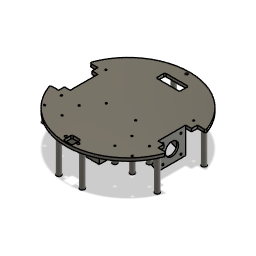
podvozek9_line_follow v3 (Autodesk Fusion 360 design; units mm, degrees)
Autodesk Fusion 360 part; units mm, degrees
sketch "zakladna" plane through (0, 0, 0) normal (0, 1, 0) x (1, 0, 0)
  line L0 (-40.0372, -23.4927) -> (-85, -23.4927)
  line L1 (39.9628, -23.4927) -> (85, -23.4927)
  line L2 (-85, 23.5073) -> (-40.0372, 23.5073)
  line L3 (85, 23.5073) -> (39.9628, 23.5073)
  line L4 (1.75, 0) -> (22.5, 0)
  line L5 (-96.7123, 33.4364) -> (-85, 33.4364)
  line L6 (-85, 33.4364) -> (-85, 23.5073)
  line L7 (-96.7154, -33.4277) -> (-85, -33.4277)
  line L8 (-85, -33.4277) -> (-85, -23.4927)
  line L9 (96.7154, -33.4277) -> (85, -33.4277)
  line L10 (85, -33.4277) -> (85, -23.4927)
  line L11 (96.7123, 33.4364) -> (85, 33.4364)
  line L12 (85, 33.4364) -> (85, 23.5073)
  arc A0 (-98.5934, -36.1156) -> (98.5934, -36.1156) centre (0, 0) ccw
  arc A1 (-96.7154, -33.4277) -> (-98.5934, -36.1156) centre (-96.7154, -35.4277) ccw
  arc A2 (-98.5902, 36.1245) -> (-96.7123, 33.4364) centre (-96.7123, 35.4364) ccw
  arc A3 (96.7123, 33.4364) -> (98.5902, 36.1245) centre (96.7123, 35.4364) ccw
  arc A4 (98.5934, -36.1156) -> (96.7154, -33.4277) centre (96.7154, -35.4277) ccw
  line L13 (0, -1.75) -> (0, -22.5)
  line L14 (39.9628, -23.4927) -> (34.9628, -23.4927)
  line L15 (34.9628, -23.4927) -> (34.9628, 23.5073)
  line L16 (34.9628, 23.5073) -> (39.9628, 23.5073)
  line L17 (-40.0372, -23.4927) -> (-35.0372, -23.4927)
  line L18 (-35.0372, -23.4927) -> (-35.0372, 23.5073)
  line L19 (-35.0372, 23.5073) -> (-40.0372, 23.5073)
  line L20 (0, -20) -> (0, -2.5)
  line L21 (2.5, 0) -> (20, 0)
  line L22 (0, 105) -> (0, -105) construction
  line L23 (-105, 0) -> (104.2756, 0.0073) construction
  line L24 (-40, -12.9977) -> (44.2998, -12.9948) construction
  circle A5 centre (-25, -11.9963) radius 1.4
  circle A6 centre (-75, 37.0037) radius 1.4
  circle A7 centre (25, -11.9963) radius 1.4
  circle A8 centre (75, 37.0037) radius 1.4
  line L25 (-20, 83.0037) -> (20, 83.0037)
  line L26 (20, 83.0037) -> (20, 68.0037)
  line L27 (20, 68.0037) -> (-20, 68.0037)
  line L28 (-20, 68.0037) -> (-20, 83.0037)
  circle A9 centre (-10.5, -95.4967) radius 2.1
  circle A10 centre (10.5, -95.4967) radius 2.1
  line L29 (-5.5, -87.9967) -> (5.5, -87.9967)
  line L30 (7.5, -89.9967) -> (7.5, -100.9967)
  line L31 (5.5, -102.9967) -> (-5.5, -102.9967)
  line L32 (-7.5, -100.9967) -> (-7.5, -89.9967)
  line L33 (-10.5, -95.4967) -> (10.5, -95.4967) construction
  arc A11 (-5.5, -87.9967) -> (-7.5, -89.9967) centre (-5.5, -89.9967) ccw
  arc A12 (7.5, -89.9967) -> (5.5, -87.9967) centre (5.5, -89.9967) ccw
  arc A13 (5.5, -102.9967) -> (7.5, -100.9967) centre (5.5, -100.9967) ccw
  arc A14 (-7.5, -100.9967) -> (-5.5, -102.9967) centre (-5.5, -100.9967) ccw
  arc A15 (98.5902, 36.1245) -> (15, 103.923) centre (0, 0) ccw
  arc A16 (-15, 103.923) -> (-98.5902, 36.1245) centre (0, 0) ccw
  line L34 (75, -38.4927) -> (45, -38.4927) construction
  line L35 (45, -38.4927) -> (45, -67.4927) construction
  line L36 (45, -67.4927) -> (75, -67.4927) construction
  line L37 (75, -67.4927) -> (75, -38.4927) construction
  circle A17 centre (45, -38.4927) radius 1.45
  circle A18 centre (75, -38.4927) radius 1.45
  circle A19 centre (45, -67.4927) radius 1.45
  circle A20 centre (75, -67.4927) radius 1.45
  circle A21 centre (-45, -38.4927) radius 1.45
  circle A22 centre (-75, -38.4927) radius 1.45
  circle A23 centre (-75, -67.4927) radius 1.45
  circle A24 centre (-45, -67.4927) radius 1.45
  line L38 (34.9628, -23.4927) -> (74.9628, -23.4927)
  line L39 (74.9628, -23.4927) -> (74.9628, 23.5073)
  line L40 (74.9628, 23.5073) -> (34.9628, 23.5073)
  line L41 (34.9628, 23.5073) -> (34.9628, -23.4927)
  line L42 (-35.0372, -23.4927) -> (-75.0372, -23.4927)
  line L43 (-75.0372, -23.4927) -> (-75.0372, 23.5073)
  line L44 (-75.0372, 23.5073) -> (-35.0372, 23.5073)
  line L45 (-35.0372, 23.5073) -> (-35.0372, -23.4927)
  arc A25 (15, 103.923) -> (-15, 103.923) centre (0, 0) ccw
  circle A26 centre (0, 100) radius 2.1
  point P0 (-82.0372, 22.8073)
  point P1 (-17.0372, -22.7927)
  point P2 (-0.0372, 0.0073)
  point P3 (81.9628, 22.8073)
  point P4 (-82.0372, -22.7927)
  point P5 (16.9628, 22.8073)
  point P6 (16.9628, 27.0073)
  point P7 (-17.0372, 27.0073)
  point P8 (81.9628, -22.7927)
  point P9 (16.9628, -22.7927)
  point P10 (16.9628, -26.9927)
  point P11 (-7.5, -87.9967)
  point P12 (7.5, -87.9967)
  point P13 (-7.5, -102.9967)
  dimension "d87" = 210
  dimension "d134" = 2
  dimension "d135" = 2
  dimension "d136" = 2
  dimension "d137" = 2
  dimension "d197" = 47
  dimension "d199" = 47
  dimension "d205" = 13
  dimension "d206" = 2.8
  dimension "d207" = 2.8
  dimension "d208" = 49
  dimension "d209" = 50
  dimension "d210" = 40
  dimension "d211" = 15
  dimension "d212" = 80
  dimension "d216" = 4.2
  dimension "d217" = 10.5
  dimension "d220" = 15
  dimension "d221" = 15
  dimension "d222" = 2
  dimension "d223" = 2
  dimension "d224" = 2
  dimension "d225" = 2
  dimension "d232" = 95.5
  dimension "d237" = 25
  dimension "d258" = 30
  dimension "d259" = 29
  dimension "d260" = 2.9
  dimension "d261" = 2.9
  dimension "d262" = 2.9
  dimension "d263" = 2.9
  dimension "d264" = 45
  dimension "d265" = 15
  dimension "d266" = 40
  dimension "d267" = 40
  dimension "d268" = 47
  dimension "d298" = 4.2
  dimension "d299" = 5
  constraint horizontal L2
  constraint horizontal L0
  constraint horizontal L3
  constraint horizontal L1
  constraint horizontal L5
  constraint vertical L6
  constraint horizontal L7
  constraint vertical L8
  constraint horizontal L9
  constraint vertical L10
  constraint horizontal L11
  constraint vertical L12
  constraint coincident A0.centre A15.centre
  constraint concentric A0 A15
  constraint tangent A0 A1
  constraint tangent L7 A1
  constraint tangent A2 A15
  constraint tangent L5 A2
  constraint tangent L11 A3
  constraint tangent A3 A15
  constraint tangent L9 A4
  constraint tangent A0 A4
  constraint horizontal L14
  constraint vertical L15
  constraint horizontal L16
  constraint horizontal L17
  constraint vertical L18
  constraint horizontal L19
  constraint midpoint A0 L22.end
  constraint parallel L20 L22
  constraint parallel L23 L24
  constraint symmetric L22 A5 A7
  constraint symmetric L22 A6 A8
  constraint horizontal L25
  constraint vertical L26
  constraint horizontal L27
  constraint vertical L28
  constraint symmetric L22 L26 L28
  constraint symmetric L22 A9 A10
  constraint horizontal L29
  constraint vertical L30
  constraint horizontal L31
  constraint vertical L32
  constraint symmetric L22 L30 L32
  constraint coincident A9.centre L33.start
  constraint coincident A10.centre L33.end
  constraint symmetric L29 L31 L33
  constraint coincident P11 L29
  constraint coincident P11 L32
  constraint tangent L29 A11
  constraint tangent L32 A11
  constraint coincident P12 L29
  constraint coincident P12 L30
  constraint tangent L29 A12
  constraint tangent L30 A12
  constraint tangent L30 A13
  constraint tangent L31 A13
  constraint coincident P13 L31
  constraint coincident P13 L32
  constraint tangent L31 A14
  constraint tangent L32 A14
  constraint concentric A15 A16
  constraint coincident L22.start A15
  constraint horizontal L34
  constraint vertical L35
  constraint horizontal L36
  constraint vertical L37
  constraint coincident L34.end L35.start
  constraint coincident L34.start L37.end
  constraint coincident L35.end L36.start
  constraint coincident L36.end L37.start
  constraint symmetric L22 A17 A21
  constraint symmetric L22 A18 A22
  constraint symmetric L22 A19 A24
  constraint symmetric L22 A20 A23
  constraint horizontal L38
  constraint vertical L39
  constraint horizontal L40
  constraint vertical L41
  constraint horizontal L42
  constraint vertical L43
  constraint horizontal L44
  constraint vertical L45
  constraint coincident L22.start A25
  constraint coincident L22 A26.centre
  measures "d87" diameter of A15
  measures "d134" radius of A1
  measures "d135" radius of A2
  measures "d136" radius of A3
  measures "d137" radius of A4
  measures "d197" distance of L1.start L3.end
  measures "d199" distance of L0.start L2.end
  measures "d205" distance of L23 L24
  measures "d206" diameter of A5
  measures "d207" diameter of A6
  measures "d208" vertical distance of A5.centre A6.centre
  measures "d209" horizontal distance of A5.centre A6.centre
  measures "d210" distance of L25.start L25.end
  measures "d211" distance of L25.start L27.end
  measures "d212" distance of A7.centre L27
  measures "d216" diameter of A9
  measures "d217" distance of L22 A9.centre
  measures "d220" distance of P11 P12
  measures "d221" distance of P11 P13
  measures "d222" radius of A11
  measures "d223" radius of A12
  measures "d224" radius of A13
  measures "d225" radius of A14
  measures "d232" distance of L23 A9.centre
  measures "d237" distance of L22 A5.centre
  measures "d258" distance of L34.start L34.end
  measures "d259" distance of L34.start L36.end
  measures "d260" diameter of A17
  measures "d261" diameter of A18
  measures "d262" diameter of A19
  measures "d263" diameter of A20
  measures "d264" distance of L22 L34.end
  measures "d265" distance of L1 L34.end
  measures "d266" distance of L14.end L38.end
  measures "d267" distance of L17.end L42.end
  measures "d268" distance of L17.end L18.end
  measures "d298" diameter of A26
  measures "d299" distance of L22.start A26.centre
extrude "Extrude23" add sketch "zakladna" along normal blind 5 contours L0 L1 L2 L3 L5 L6 L7 L8 L9 L10 L11 L12 A0 A1 A2 A3 A4 L14 L15 L16 L17 L18 L19 A15 A16 L38 L40 L41 L42 L44 L45 A25
sketch "beterka" plane through (0, 0, 0) normal (0, 1, 0) x (1, 0, 0)
  line L0 (-36, -25) -> (36, -25)
  line L1 (36, -25) -> (36, -85)
  line L2 (36, -85) -> (-36, -85)
  line L3 (-36, -85) -> (-36, -25)
  line L4 (0, 105) -> (0, -105)
  line L5 (2.5, 0) -> (20, 0)
  line L6 (37.5, -86.5) -> (-37.5, -86.5)
  line L7 (-37.5, -86.5) -> (-37.5, -23.5)
  line L8 (-37.5, -23.5) -> (37.5, -23.5)
  line L9 (37.5, -23.5) -> (37.5, -86.5)
  dimension "d228" = 72
  dimension "d229" = 60
  dimension "d230" = 25
  dimension "d231" = -1.5
  constraint horizontal L0
  constraint vertical L1
  constraint horizontal L2
  constraint vertical L3
  constraint symmetric L1 L3 L4
  measures "d228" distance of L0.start L0.end
  measures "d229" distance of L0.start L2.end
  measures "d230" distance of L0 L5
extrude "Extrude25" add sketch "beterka" against normal blind 17 contours L0 L2 L3 L4 L6 L7 L8 | L0 L1 L2 L4 L6 L8 L9
sketch "zvyseni" plane through (0, 0, 0) normal (0, 1, 0) x (1, 0, 0)
  circle A0 centre (25, -11.9963) radius 4
  circle A1 centre (25, -11.9963) radius 1.4
  circle A2 centre (-25, -11.9963) radius 1.4
  circle A3 centre (-25, -11.9963) radius 4
  circle A4 centre (75, 37.0037) radius 1.4
  circle A5 centre (75, 37.0037) radius 4
  circle A6 centre (-75, 37.0037) radius 1.4
  circle A7 centre (-75, 37.0037) radius 4
  line L0 (5, 90) -> (-5, 90)
  line L1 (-5, 90) -> (-5, 85)
  line L2 (-5, 85) -> (5, 85)
  line L3 (5, 85) -> (5, 90)
  point P0 (25, -11.9963)
  point P1 (-25, -11.9963)
  point P2 (75, 37.0037)
  point P3 (-75, 37.0037)
  dimension "d250" = 8
  dimension "d251" = 8
  dimension "d252" = 8
  dimension "d253" = 8
  constraint coincident P0 A0.centre
  constraint coincident P1 A2.centre
  constraint coincident P2 A4.centre
  constraint concentric A4 A5
  constraint coincident P3 A6.centre
  constraint concentric A6 A7
  constraint horizontal L0
  constraint vertical L1
  constraint horizontal L2
  constraint vertical L3
  measures "d250" diameter of A0
  measures "d251" diameter of A3
  measures "d252" diameter of A5
  measures "d253" diameter of A7
extrude "Extrude26" add sketch "zvyseni" against normal blind 1.6
sketch " motory_podklad" plane through (0, 5, 0) normal (0, 1, 0) x (-1, 0, 0)
  circle A0 centre (-45, 67.4927) radius 1.45
  circle A1 centre (-10.5, 95.4967) radius 2.1
  circle A2 centre (-75, 38.4927) radius 1.45
  arc A3 (5.5, 87.9967) -> (7.5, 89.9967) centre (5.5, 89.9967) ccw
  line L0 (5.5, 87.9967) -> (-5.5, 87.9967)
  arc A4 (-7.5, 89.9967) -> (-5.5, 87.9967) centre (-5.5, 89.9967) ccw
  line L1 (-7.5, 89.9967) -> (-7.5, 100.9967)
  arc A5 (-5.5, 102.9967) -> (-7.5, 100.9967) centre (-5.5, 100.9967) ccw
  line L2 (-5.5, 102.9967) -> (5.5, 102.9967)
  arc A6 (7.5, 100.9967) -> (5.5, 102.9967) centre (5.5, 100.9967) ccw
  line L3 (7.5, 100.9967) -> (7.5, 89.9967)
  circle A7 centre (-75, -37.0037) radius 1.4
  circle A8 centre (25, 11.9963) radius 1.4
  circle A9 centre (-45, 38.4927) radius 1.45
  circle A10 centre (45, 67.4927) radius 1.45
  circle A11 centre (75, -37.0037) radius 1.4
  circle A12 centre (75, 67.4927) radius 1.45
  line L4 (-20, -68.0037) -> (20, -68.0037)
  line L5 (20, -68.0037) -> (20, -83.0037)
  line L6 (20, -83.0037) -> (-20, -83.0037)
  line L7 (-20, -83.0037) -> (-20, -68.0037)
  circle A13 centre (10.5, 95.4967) radius 2.1
  circle A14 centre (45, 38.4927) radius 1.45
  circle A15 centre (75, 38.4927) radius 1.45
  circle A16 centre (-25, 11.9963) radius 1.4
  circle A17 centre (-75, 67.4927) radius 1.45
  arc A18 (-96.7123, -33.4364) -> (-98.5902, -36.1245) centre (-96.7123, -35.4364) ccw
  arc A19 (-98.5902, -36.1245) -> (98.5902, -36.1245) centre (0, 0) ccw
  arc A20 (98.5902, -36.1245) -> (96.7123, -33.4364) centre (96.7123, -35.4364) ccw
  line L8 (96.7123, -33.4364) -> (85, -33.4364)
  line L9 (85, -33.4364) -> (85, -23.5073)
  line L10 (85, -23.5073) -> (35.0372, -23.5073)
  line L11 (35.0372, -23.5073) -> (35.0372, 23.4927)
  line L12 (35.0372, 23.4927) -> (85, 23.4927)
  line L13 (85, 23.4927) -> (85, 33.4277)
  line L14 (85, 33.4277) -> (96.7154, 33.4277)
  arc A21 (96.7154, 33.4277) -> (98.5934, 36.1156) centre (96.7154, 35.4277) ccw
  arc A22 (98.5934, 36.1156) -> (-98.5934, 36.1156) centre (0, 0) ccw
  arc A23 (-98.5934, 36.1156) -> (-96.7154, 33.4277) centre (-96.7154, 35.4277) ccw
  line L15 (-96.7154, 33.4277) -> (-85, 33.4277)
  line L16 (-85, 33.4277) -> (-85, 23.4927)
  line L17 (-85, 23.4927) -> (-34.9628, 23.4927)
  line L18 (-34.9628, 23.4927) -> (-34.9628, -23.5073)
  line L19 (-34.9628, -23.5073) -> (-85, -23.5073)
  line L20 (-85, -23.5073) -> (-85, -33.4364)
  line L21 (-85, -33.4364) -> (-96.7123, -33.4364)
  line L22 (75.0372, -23.5073) -> (35.0372, -23.5073)
  line L23 (35.0372, -23.5073) -> (35.0372, 23.4927)
  line L24 (35.0372, 23.4927) -> (75.0372, 23.4927)
  line L25 (75.0372, 23.4927) -> (75.0372, -23.5073)
  line L26 (-34.9628, -23.5073) -> (-74.9628, -23.5073)
  line L27 (-74.9628, -23.5073) -> (-74.9628, 23.4927)
  line L28 (-74.9628, 23.4927) -> (-34.9628, 23.4927)
  line L29 (-34.9628, 23.4927) -> (-34.9628, -23.5073)
  line L30 (75.0372, 23.4927) -> (75.0372, -23.5073)
  line L31 (35.0372, 23.4927) -> (75.0372, 23.4927)
  circle A24 centre (0, -100) radius 2.1
  point P0 (75.0372, -23.5073)
  point P1 (-74.9628, 23.4927)
  dimension "d271" = 47
  dimension "d272" = 40
  constraint horizontal L22
  constraint vertical L23
  constraint horizontal L24
  constraint vertical L25
  constraint coincident L11.end L12.start
  constraint coincident P0 L22.start
  constraint horizontal L26
  constraint vertical L27
  constraint horizontal L28
  constraint vertical L29
  constraint coincident P1 L27.end
  constraint coincident L18.end L19.start
  measures "d271" distance of L24.end P0
  measures "d272" distance of L24.end L11.end
extrude "Extrude27" add sketch " motory_podklad" against normal blind 45 contours L17 L18 L19 L26 L27 L28 L29 | L10 L11 L12 L22 L23 L24 L25 L30 L31
sketch "motory_kapsa" plane through (0, -40, 0) normal (0, -1, 0) x (1, 0, 0)
  line L0 (-35.0372, 23.4927) -> (-75.0372, 23.4927)
  line L1 (-75.0372, 23.4927) -> (-75.0372, -23.5073)
  line L2 (-75.0372, -23.5073) -> (-35.0372, -23.5073)
  line L3 (-35.0372, -23.5073) -> (-35.0372, 23.4927)
  line L4 (-35.0372, 21.4927) -> (-72.0372, 21.4927)
  line L5 (-72.0372, 21.4927) -> (-72.0372, -21.5073)
  line L6 (-72.0372, -21.5073) -> (-35.0372, -21.5073)
  line L7 (-35.0372, -21.5073) -> (-35.0372, 21.4927)
  line L8 (0, -105) -> (0, 105)
  line L9 (34.9628, 21.4927) -> (71.9628, 21.4927)
  line L10 (71.9628, 21.4927) -> (71.9628, -21.5073)
  line L11 (71.9628, -21.5073) -> (34.9628, -21.5073)
  line L12 (34.9628, -21.5073) -> (34.9628, 21.4927)
  line L13 (34.9628, -23.5073) -> (34.9628, 23.4927)
  line L14 (74.9628, 23.4927) -> (34.9628, 23.4927)
  dimension "d273" = 37
  dimension "d274" = 43
  dimension "d275" = 2
  dimension "d278" = 37
  dimension "d279" = 43
  dimension "d280" = 2
  constraint horizontal L4
  constraint vertical L5
  constraint horizontal L6
  constraint vertical L7
  constraint coincident L3 L4.start
  constraint horizontal L9
  constraint vertical L10
  constraint horizontal L11
  constraint vertical L12
  constraint coincident L9.start L13
  measures "d273" distance of L4.start L4.end
  measures "d274" distance of L4.start L6.end
  measures "d275" distance of L0 L4
  measures "d278" distance of L9.start L9.end
  measures "d279" distance of L9.start L11.end
  measures "d280" distance of L9 L14
extrude "Extrude29" cut sketch "motory_kapsa" against normal blind 43 contours L3 L4 L5 L6 L7 | L9 L10 L11 L12 L13
sketch "motory_diry" plane through (71.9628, 0, 0) normal (-1, 0, 0) x (0, 0, 1)
  line L0 (-21.5073, -40) -> (21.4927, -40)
  line L1 (21.4927, -40) -> (21.4927, 3)
  line L2 (21.4927, 3) -> (-21.5073, 3)
  line L3 (-21.5073, 3) -> (-21.5073, -40)
  line L4 (0, -26.6328) -> (0, -8.6328) construction
  line L5 (23, -18.5) -> (-28, -18.5) construction
  circle A0 centre (0, -18.5) radius 11.25
  circle A1 centre (15.5, -34) radius 1.6
  circle A2 centre (-15.5, -34) radius 1.6
  circle A3 centre (15.5, -3) radius 1.6
  circle A4 centre (-15.5, -3) radius 1.6
  dimension "d283" = 43
  dimension "d284" = 43
  dimension "d285" = 21.5
  dimension "d286" = 22.5
  dimension "d287" = 3.2
  dimension "d288" = 15.5
  dimension "d289" = 15.5
  constraint vertical L4
  constraint perpendicular L3 L5
  constraint coincident L4 A0.centre
  constraint coincident L5 A0.centre
  constraint symmetric L4 A1 A2
  constraint symmetric L5 A1 A3
  constraint symmetric L5 A2 A4
  measures "d283" distance of L0.end L1.end
  measures "d284" distance of L0.start L0.end
  measures "d285" distance of L2 L5
  measures "d286" diameter of A0
  measures "d287" diameter of A1
  measures "d288" distance of L4 A1.centre
  measures "d289" distance of L5 A1.centre
extrude "Extrude30" cut sketch "motory_diry" along normal through all and the other way through all contours A0 | A1 | A2 | A3 | A4
sketch "snizeni_motory" plane through (0, 0, 23.4927) normal (0, 0, 1) x (1, 0, 0)
  line L0 (74.9628, 0) -> (34.9628, 0)
  line L1 (34.9628, 0) -> (34.9628, -40)
  line L2 (34.9628, -40) -> (74.9628, -40)
  line L3 (74.9628, -40) -> (74.9628, 0)
  line L4 (71.9628, -40) -> (39.9159, -25.4626)
  line L5 (39.9159, -25.4626) -> (39.9159, -17)
  line L6 (37.5, -17) -> (-37.5, -17)
  line L7 (39.9159, -17) -> (0, -17)
  line L8 (0, -40) -> (71.9628, -40)
  line L9 (0, 2.5) -> (0, 20)
  line L10 (-71.9628, -40) -> (-39.9159, -25.4626)
  line L11 (0, -40) -> (-71.9628, -40)
  line L12 (-39.9159, -25.4626) -> (-39.9159, -17)
  line L13 (-39.9159, -17) -> (0, -17)
  point P0 (71.9628, -40)
  point P1 (71.9628, -40)
  constraint coincident P1 P0
  constraint perpendicular L2 L5
  constraint midpoint L6 L7.end
  constraint symmetric P1 L9 L10.start
  constraint symmetric L4.end L9 L10.end
  constraint symmetric L5.end L9 L12.end
  constraint symmetric L7.end L9 L13.end
  constraint symmetric L8.start L9 L11.start
extrude "Extrude32" cut sketch "snizeni_motory" against normal blind 53 contours L1 L2 L4 L5 L6 L7 L8 | L1 L6 L7 L8 L10 L11 L12 L13
chamfer "Chamfer1" distance 3 angle 45 2 edges at (34.9628, 0, -0.0073) (-35.0372, 0, -0.0073)
sketch "Sketch21" plane through (0, 0, 0) normal (0, -1, 0) x (1, 0, 0)
  line L0 (-37.5, 23.5) -> (-37.5, 86.5)
  line L1 (-37.5, 86.5) -> (37.5, 86.5)
  line L2 (37.5, 86.5) -> (37.5, 23.5)
  line L3 (37.5, 23.5) -> (-37.5, 23.5)
  circle A0 centre (0, -100) radius 2.1
  circle A1 centre (75, 67.4927) radius 1.45
  circle A2 centre (-45, 38.4927) radius 1.45
  line L4 (-20, -68.0037) -> (20, -68.0037)
  line L5 (20, -68.0037) -> (20, -83.0037)
  line L6 (20, -83.0037) -> (-20, -83.0037)
  line L7 (-20, -83.0037) -> (-20, -68.0037)
  circle A3 centre (75, 38.4927) radius 1.45
  arc A4 (-7.5, 89.9967) -> (-5.5, 87.9967) centre (-5.5, 89.9967) ccw
  line L8 (-7.5, 89.9967) -> (-7.5, 100.9967)
  arc A5 (-5.5, 102.9967) -> (-7.5, 100.9967) centre (-5.5, 100.9967) ccw
  line L9 (-5.5, 102.9967) -> (5.5, 102.9967)
  arc A6 (7.5, 100.9967) -> (5.5, 102.9967) centre (5.5, 100.9967) ccw
  line L10 (7.5, 100.9967) -> (7.5, 89.9967)
  arc A7 (5.5, 87.9967) -> (7.5, 89.9967) centre (5.5, 89.9967) ccw
  line L11 (5.5, 87.9967) -> (-5.5, 87.9967)
  circle A8 centre (-75, 67.4927) radius 1.45
  circle A9 centre (45, 67.4927) radius 1.45
  circle A10 centre (-10.5, 95.4967) radius 2.1
  circle A11 centre (10.5, 95.4967) radius 2.1
  circle A12 centre (-45, 67.4927) radius 1.45
  circle A13 centre (-75, 38.4927) radius 1.45
  circle A14 centre (45, 38.4927) radius 1.45
  circle A15 centre (-25, 11.9963) radius 4
  circle A16 centre (75, -37.0037) radius 4
  circle A17 centre (25, 11.9963) radius 4
  circle A18 centre (-75, -37.0037) radius 4
  line L12 (5, -90) -> (-5, -90)
  line L13 (-5, -90) -> (-5, -85)
  line L14 (-5, -85) -> (5, -85)
  line L15 (5, -85) -> (5, -90)
  line L16 (-35.0372, 21.4927) -> (-32.0372, 21.4927)
  line L17 (-32.0372, 21.4927) -> (-32.0372, -21.5073)
  line L18 (-32.0372, -21.5073) -> (-35.0372, -21.5073)
  line L19 (-35.0372, -21.5073) -> (-35.0372, -23.5073)
  line L20 (-35.0372, -23.5073) -> (-75.0372, -23.5073)
  line L21 (-75.0372, -23.5073) -> (-85, -23.5073)
  line L22 (-85, -23.5073) -> (-85, -33.4364)
  line L23 (-85, -33.4364) -> (-96.7123, -33.4364)
  arc A19 (-96.7123, -33.4364) -> (-98.5902, -36.1245) centre (-96.7123, -35.4364) ccw
  arc A20 (-98.5902, -36.1245) -> (98.5902, -36.1245) centre (0, 0) ccw
  arc A21 (98.5902, -36.1245) -> (96.7123, -33.4364) centre (96.7123, -35.4364) ccw
  line L24 (96.7123, -33.4364) -> (85, -33.4364)
  line L25 (85, -33.4364) -> (85, -23.5073)
  line L26 (85, -23.5073) -> (74.9628, -23.5073)
  line L27 (74.9628, -23.5073) -> (34.9628, -23.5073)
  line L28 (34.9628, -23.5073) -> (34.9628, -21.5073)
  line L29 (34.9628, -21.5073) -> (31.9628, -21.5073)
  line L30 (31.9628, -21.5073) -> (31.9628, 21.4927)
  line L31 (31.9628, 21.4927) -> (34.9628, 21.4927)
  line L32 (34.9628, 21.4927) -> (34.9628, 23.4927)
  line L33 (34.9628, 23.4927) -> (74.9628, 23.4927)
  line L34 (74.9628, 23.4927) -> (85, 23.4927)
  line L35 (85, 23.4927) -> (85, 33.4277)
  line L36 (85, 33.4277) -> (96.7154, 33.4277)
  arc A22 (96.7154, 33.4277) -> (98.5934, 36.1156) centre (96.7154, 35.4277) ccw
  arc A23 (98.5934, 36.1156) -> (-98.5934, 36.1156) centre (0, 0) ccw
  arc A24 (-98.5934, 36.1156) -> (-96.7154, 33.4277) centre (-96.7154, 35.4277) ccw
  line L37 (-96.7154, 33.4277) -> (-85, 33.4277)
  line L38 (-85, 33.4277) -> (-85, 23.4927)
  line L39 (-85, 23.4927) -> (-75.0372, 23.4927)
  line L40 (-75.0372, 23.4927) -> (-35.0372, 23.4927)
  line L41 (-35.0372, 23.4927) -> (-35.0372, 21.4927)
  circle A25 centre (-75, 38.4927) radius 4
  circle A26 centre (-45, 38.4927) radius 4
  circle A27 centre (-45, 67.4927) radius 4
  circle A28 centre (-75, 67.4927) radius 4
  circle A29 centre (-75, 67.4927) radius 1.45
  circle A30 centre (-45, 67.4927) radius 1.45
  circle A31 centre (-45, 38.4927) radius 1.45
  circle A32 centre (-75, 38.4927) radius 1.45
  circle A33 centre (45, 67.4927) radius 4
  circle A34 centre (45, 38.4927) radius 4
  circle A35 centre (75, 38.4927) radius 4
  circle A36 centre (75, 67.4927) radius 4
  circle A37 centre (45, 38.4927) radius 1.45
  circle A38 centre (75, 38.4927) radius 1.45
  circle A39 centre (75, 67.4927) radius 1.45
  circle A40 centre (45, 67.4927) radius 1.45
  dimension "d300" = 8
  dimension "d301" = 8
  dimension "d302" = 8
  dimension "d303" = 8
  dimension "d304" = 8
  dimension "d305" = 8
  dimension "d306" = 8
  dimension "d307" = 8
  constraint concentric A13 A25
  constraint concentric A2 A26
  constraint concentric A12 A27
  constraint concentric A8 A28
  constraint concentric A9 A33
  constraint concentric A14 A34
  constraint concentric A3 A35
  constraint concentric A1 A36
  measures "d300" diameter of A25
  measures "d301" diameter of A26
  measures "d302" diameter of A27
  measures "d303" diameter of A28
  measures "d304" diameter of A33
  measures "d305" diameter of A34
  measures "d306" diameter of A35
  measures "d307" diameter of A36
extrude "Extrude33" add sketch "Sketch21" along normal blind 20 contours A25 | A26 | A27 | A28 | A33 | A34 | A35 | A36
fillet "Fillet4" radius 2 4 edges at (20, 2.5, -68.0037) (-20, 2.5, -68.0037) (20, 2.5, -83.0037) (-20, 2.5, -83.0037)
sketch "drzaky_horniho_patra" plane through (0, 0, 0) normal (0, -1, 0) x (1, 0, 0)
  circle A0 centre (-75, 38.4927) radius 4
  circle A1 centre (75, 67.4927) radius 4
  circle A2 centre (-75, 67.4927) radius 4
  circle A3 centre (75, 38.4927) radius 4
  circle A4 centre (-45, 38.4927) radius 4
  circle A5 centre (45, 67.4927) radius 4
  circle A6 centre (-45, 67.4927) radius 4
  circle A7 centre (45, 38.4927) radius 4
  line L0 (-37.5, 23.5) -> (-37.5, 86.5)
  line L1 (-37.5, 86.5) -> (37.5, 86.5)
  line L2 (37.5, 86.5) -> (37.5, 23.5)
  line L3 (37.5, 23.5) -> (-37.5, 23.5)
  circle A8 centre (-10.5, 95.4967) radius 2.1
  circle A9 centre (10.5, 95.4967) radius 2.1
  arc A10 (20, -70.0037) -> (18, -68.0037) centre (18, -70.0037) ccw
  line L4 (20, -70.0037) -> (20, -81.0037)
  arc A11 (18, -83.0037) -> (20, -81.0037) centre (18, -81.0037) ccw
  line L5 (18, -83.0037) -> (-18, -83.0037)
  arc A12 (-20, -81.0037) -> (-18, -83.0037) centre (-18, -81.0037) ccw
  line L6 (-20, -81.0037) -> (-20, -70.0037)
  arc A13 (-18, -68.0037) -> (-20, -70.0037) centre (-18, -70.0037) ccw
  line L7 (-18, -68.0037) -> (18, -68.0037)
  circle A14 centre (0, -100) radius 2.1
  arc A15 (-7.5, 89.9967) -> (-5.5, 87.9967) centre (-5.5, 89.9967) ccw
  line L8 (-7.5, 89.9967) -> (-7.5, 100.9967)
  arc A16 (-5.5, 102.9967) -> (-7.5, 100.9967) centre (-5.5, 100.9967) ccw
  line L9 (-5.5, 102.9967) -> (5.5, 102.9967)
  arc A17 (7.5, 100.9967) -> (5.5, 102.9967) centre (5.5, 100.9967) ccw
  line L10 (7.5, 100.9967) -> (7.5, 89.9967)
  arc A18 (5.5, 87.9967) -> (7.5, 89.9967) centre (5.5, 89.9967) ccw
  line L11 (5.5, 87.9967) -> (-5.5, 87.9967)
  circle A19 centre (-25, 11.9963) radius 4
  circle A20 centre (75, -37.0037) radius 4
  circle A21 centre (25, 11.9963) radius 4
  circle A22 centre (-75, -37.0037) radius 4
  line L12 (5, -90) -> (-5, -90)
  line L13 (-5, -90) -> (-5, -85)
  line L14 (-5, -85) -> (5, -85)
  line L15 (5, -85) -> (5, -90)
  line L16 (-35.0372, 21.4927) -> (-32.0372, 21.4927)
  line L17 (-32.0372, 21.4927) -> (-32.0372, -21.5073)
  line L18 (-32.0372, -21.5073) -> (-35.0372, -21.5073)
  line L19 (-35.0372, -21.5073) -> (-35.0372, -23.5073)
  line L20 (-35.0372, -23.5073) -> (-75.0372, -23.5073)
  line L21 (-75.0372, -23.5073) -> (-85, -23.5073)
  line L22 (-85, -23.5073) -> (-85, -33.4364)
  line L23 (-85, -33.4364) -> (-96.7123, -33.4364)
  arc A23 (-96.7123, -33.4364) -> (-98.5902, -36.1245) centre (-96.7123, -35.4364) ccw
  arc A24 (-98.5902, -36.1245) -> (98.5902, -36.1245) centre (0, 0) ccw
  arc A25 (98.5902, -36.1245) -> (96.7123, -33.4364) centre (96.7123, -35.4364) ccw
  line L24 (96.7123, -33.4364) -> (85, -33.4364)
  line L25 (85, -33.4364) -> (85, -23.5073)
  line L26 (85, -23.5073) -> (74.9628, -23.5073)
  line L27 (74.9628, -23.5073) -> (34.9628, -23.5073)
  line L28 (34.9628, -23.5073) -> (34.9628, -21.5073)
  line L29 (34.9628, -21.5073) -> (31.9628, -21.5073)
  line L30 (31.9628, -21.5073) -> (31.9628, 21.4927)
  line L31 (31.9628, 21.4927) -> (34.9628, 21.4927)
  line L32 (34.9628, 21.4927) -> (34.9628, 23.4927)
  line L33 (34.9628, 23.4927) -> (74.9628, 23.4927)
  line L34 (74.9628, 23.4927) -> (85, 23.4927)
  line L35 (85, 23.4927) -> (85, 33.4277)
  line L36 (85, 33.4277) -> (96.7154, 33.4277)
  arc A26 (96.7154, 33.4277) -> (98.5934, 36.1156) centre (96.7154, 35.4277) ccw
  arc A27 (98.5934, 36.1156) -> (-98.5934, 36.1156) centre (0, 0) ccw
  arc A28 (-98.5934, 36.1156) -> (-96.7154, 33.4277) centre (-96.7154, 35.4277) ccw
  line L37 (-96.7154, 33.4277) -> (-85, 33.4277)
  line L38 (-85, 33.4277) -> (-85, 23.4927)
  line L39 (-85, 23.4927) -> (-75.0372, 23.4927)
  line L40 (-75.0372, 23.4927) -> (-35.0372, 23.4927)
  line L41 (-35.0372, 23.4927) -> (-35.0372, 21.4927)
  circle A29 centre (-90, 39.9995) radius 4
  line L42 (-105, 0) -> (104.2756, -0.0073)
  circle A30 centre (-90, 39.9995) radius 1.45
  line L43 (0, -105) -> (0, 105)
  circle A31 centre (90, 39.9995) radius 4
  circle A32 centre (90, 39.9995) radius 1.45
  circle A33 centre (-90.0028, -40.0005) radius 4
  circle A34 centre (-90.0028, -40.0005) radius 1.45
  circle A35 centre (89.9972, -40.0131) radius 4
  circle A36 centre (89.9972, -40.0131) radius 1.45
  circle A37 centre (20, -98.0044) radius 4
  circle A38 centre (20, -98.0044) radius 1.45
  circle A39 centre (-20, -98.0044) radius 4
  circle A40 centre (-20, -98.0044) radius 1.45
  circle A41 centre (-19.9932, 97.9984) radius 4
  circle A42 centre (20.0068, 97.9956) radius 4
  circle A43 centre (20.0068, 97.9956) radius 1.45
  circle A44 centre (-19.9932, 97.9984) radius 1.45
  dimension "d312" = 8
  dimension "d313" = 40
  dimension "d314" = 2.9
  dimension "d315" = 8
  dimension "d316" = 20
  dimension "d317" = 98
  dimension "d318" = 2.9
  constraint concentric A29 A30
  constraint symmetric A29 L43 A31
  constraint symmetric A30 L43 A32
  constraint symmetric A29 L42 A33
  constraint symmetric L42 A30 A34
  constraint symmetric L42 A31 A35
  constraint symmetric L42 A32 A36
  constraint concentric A37 A38
  constraint symmetric L43 A37 A39
  constraint symmetric L43 A38 A40
  constraint symmetric L42 A37 A42
  constraint symmetric L42 A38 A43
  constraint symmetric L42 A39 A41
  constraint symmetric L42 A40 A44
  measures "d312" diameter of A29
  measures "d313" distance of A29.centre L42
  measures "d314" diameter of A30
  measures "d315" diameter of A37
  measures "d316" distance of L43 A37.centre
  measures "d317" distance of L42 A37.centre
  measures "d318" diameter of A38
extrude "Extrude34" add sketch "drzaky_horniho_patra" along normal blind 55 contours A29 | A31 | A33 | A35 | A37 | A39 | A41 | A42
equation "d285 = ( 43 / 2 ) * 1 mm"
